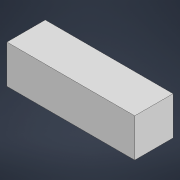
# Autodesk Inventor part: Ultrasonic Locking Pin
Saved by Autodesk Inventor 2022 (Build 260153000, 153)
## iProperties
Created: 2021-06-09
Part Number: Ultrasonic Locking Pin
Material: Generic
Document SubType Name: Modeling
Designer: saatvik123
Density: 1 g/cm^3
Appearance: Default
Author: saatvik123
## iProperties of the stored document Ultrasonic Locking Pin_3DPrint.ipt
Created: 2021-06-09
Part Number: Ultrasonic Locking Pin_3DPrint
Material: Generic
Document SubType Name: Modeling
Designer: saatvik123
Density: 1 g/cm^3
Appearance: Default
Author: saatvik123
Autodesk Inventor part; units mm, degrees
ref_plane "YZ Plane" through (0, 0, 0) normal (1, 0, 0) x (0, 1, 0)
ref_plane "XZ Plane" through (0, 0, 0) normal (0, 1, 0) x (-1, 0, 0)
ref_plane "XY Plane" through (0, 0, 0) normal (0, 0, 1) x (1, 0, 0)
sketch "Sketch1" plane through (0, 0, 0) normal (0, 1, 0) x (-1, 0, 0)
  line L0 (-3.175, 0.9525) -> (3.175, 0.9525)
  line L1 (3.175, 0.9525) -> (3.175, -0.9525)
  line L2 (3.175, -0.9525) -> (-3.175, -0.9525)
  line L3 (-3.175, -0.9525) -> (-3.175, 0.9525)
  line L4 (-3.175, 0.9525) -> (3.175, -0.9525) construction
  line L5 (3.175, 0.9525) -> (-3.175, -0.9525) construction
  point P0 (0, 0)
  dimension "d0" = 6.35
  dimension "d1" = 1.905
  constraints: 12 end point, 2 midpoint, 2 parallel, 1 horizontal, 1 perpendicular
  measures "d0" distance of L1.end L2.end
  measures "d1" distance of L0.end L1.end
extrude "Extrusion1" add sketch "Sketch1" along normal blind 1.905
body "Solid1"
